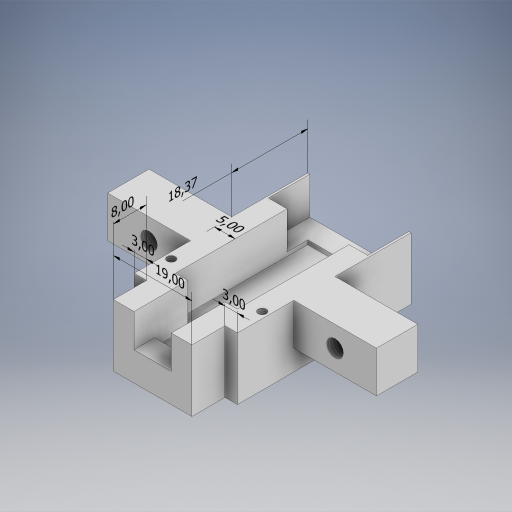
# Autodesk Inventor part: Base
Saved by Autodesk Inventor 2023 (Build 270158000, 158)
## iProperties
Created: 2024-04-01
Part Number: Base
Material: Generic
Document SubType Name: Modeling
Designer: andrew
Density: 1 g/cm^3
Appearance: Default
Author: andrew
Autodesk Inventor part; units mm, degrees
ref_plane "YZ Plane" through (0, 0, 0) normal (1, 0, 0) x (0, 1, 0)
ref_plane "XZ Plane" through (0, 0, 0) normal (0, 1, 0) x (-1, 0, 0)
ref_plane "XY Plane" through (0, 0, 0) normal (0, 0, 1) x (1, 0, 0)
sketch "Sketch1" plane through (0, 0, 0) normal (0, 1, 0) x (-1, 0, 0)
  line L0 (0, 0) -> (15, 0)
  line L1 (15, 0) -> (15, -32)
  line L2 (15, -32) -> (0, -32)
  line L3 (0, -32) -> (0, 0)
  line L4 (3, 0) -> (12, 0)
  line L5 (12, 0) -> (12, 8)
  line L6 (12, 8) -> (3, 8)
  line L7 (3, 8) -> (3, 0)
  line L8 (-5, -32) -> (-5, 5)
  line L9 (-5, 5) -> (-2, 5)
  line L10 (-2, 5) -> (-2, 13)
  line L11 (-2, 13) -> (17, 13)
  line L12 (17, 13) -> (17, 5)
  line L13 (17, 5) -> (20, 5)
  line L14 (20, 5) -> (20, -37)
  line L15 (20, -37) -> (-5, -37)
  line L16 (-5, -37) -> (-5, -32)
  line L17 (-5, -8.634) -> (-25, -8.634)
  line L18 (-25, -8.634) -> (-25, -18.634)
  line L19 (-25, -18.634) -> (-5, -18.634)
  line L20 (-5, -18.634) -> (-5, -8.634)
  line L21 (20, -18.634) -> (40, -18.634)
  line L22 (40, -18.634) -> (40, -8.634)
  line L23 (40, -8.634) -> (20, -8.634)
  line L24 (20, -8.634) -> (20, -18.634)
  dimension "d0" = 15
  dimension "d1" = 32
  dimension "d2" = 9
  dimension "d3" = 3
  dimension "d4" = 3
  dimension "d5" = 8
  dimension "d6" = 5
  dimension "d7" = 5
  dimension "d8" = 5
  dimension "d9" = 5
  dimension "d10" = 5
  dimension "d11" = 5
  dimension "d12" = 5
  dimension "d13" = 5
  dimension "d71" = 20
  dimension "d72" = 10
  dimension "d73" = 20
  dimension "d74" = 10
  constraints: 50 end point, 12 perpendicular, 8 parallel, 4 horizontal, 4 point on line, 1 vertical
  measures "d0" distance of L1.end L2.end
  measures "d1" distance of L0.end L1.end
  measures "d2" distance of L6.end L5.end
  measures "d3" distance between parallel lines of L3 L7
  measures "d4" distance between parallel lines of L1 L5
  measures "d5" distance of L4.end L5.end
  measures "d6" distance between parallel lines of L3 L8
  measures "d7" distance between parallel lines of L2 L15
  measures "d8" distance between parallel lines of L1 L14
  measures "d9" distance between parallel lines of L0 L13
  measures "d10" distance between parallel lines of L5 L12
  measures "d11" distance between parallel lines of L7 L10
  measures "d12" distance between parallel lines of L0 L9
  measures "d13" distance between parallel lines of L6 L11
  measures "d71" distance of L18.end L19.end
  measures "d72" distance of L17.end L18.end
  measures "d73" distance of L21.start L21.end
  measures "d74" distance of L21.end L22.end
extrude "Extrusion1" add sketch "Sketch1" along normal blind 10
sketch "Sketch3" plane through (5, 0, -37) normal (0, 0, -1) x (-1, 0, 0)
  line L0 (0.5, 10) -> (24.5, 10)
  line L1 (24.5, 10) -> (24.5, 1)
  line L2 (24.5, 1) -> (0.5, 1)
  line L3 (0.5, 1) -> (0.5, 10)
  line L4 (25, 0) -> (25, 10) projected
  line L5 (0, 0) -> (0, 10) projected
  line L6 (0, 0) -> (25, 0) projected
  line L7 (0, 10) -> (25, 10) projected
  point P0 (5, 0)
  point P1 (24.5, 5.5)
  dimension "d24" = 0.5
  dimension "d25" = 0.5
  dimension "d26" = 1
  dimension "d27" = 0
  constraints: 8 end point, 2 parallel, 1 horizontal, 1 midpoint, 1 perpendicular
  measures "d24" distance from line of L4 point (24.5, 5.5)
  measures "d25" distance between parallel lines of L5 L3
  measures "d26" distance between parallel lines of L6 L2
  measures "d27" distance between parallel lines of L7 L0
extrude "Extrusion3" cut sketch "Sketch3" against normal blind 10 contours L0 L1 L2 L3
sketch "Sketch4" plane through (-17, 0, 13) normal (0, 0, 1) x (1, 0, 0)
  line L0 (5, 10) -> (14, 10)
  line L1 (14, 10) -> (14, 2)
  line L2 (14, 2) -> (5, 2)
  line L3 (5, 2) -> (5, 10)
  line L4 (0, 0) -> (19, 0) projected
  line L5 (0, 10) -> (19, 10) projected
  line L6 (19, 0) -> (19, 10) projected
  line L7 (0, 0) -> (0, 10) projected
  point P0 (17, 0)
  point P1 (9.5, 0)
  dimension "d30" = 2
  dimension "d31" = 0
  dimension "d32" = 5
  dimension "d33" = 5
  constraints: 8 end point, 2 parallel, 1 horizontal, 1 midpoint, 1 perpendicular
  measures "d30" distance from line of point (9.5, 0) L2
  measures "d31" distance between parallel lines of L5 L0
  measures "d32" distance between parallel lines of L6 L1
  measures "d33" distance between parallel lines of L7 L3
extrude "Extrusion4" cut sketch "Sketch4" against normal blind 10 contours L0 L1 L2 L3
sketch "Sketch5" plane through (0, 0, 0) normal (0, -1, 0) x (1, 0, 0)
  line L0 (-17, 5) -> (-17, 13) projected
  line L1 (2, 13) -> (2, 5) projected
  line L2 (-17, 13) -> (2, 13)
  line L3 (2, 13) -> (2, 5)
  line L4 (5, 5) -> (5, -37) projected
  line L5 (2, 5) -> (5, 5)
  line L6 (5, 5) -> (5, -37)
  line L7 (-20, -37) -> (-20, 5) projected
  line L8 (5, -37) -> (-20, -37)
  line L9 (-20, -37) -> (-20, 5)
  line L10 (-20, 5) -> (-17, 5)
  point P0 (0, 0)
  constraints: 14 end point, 6 perpendicular, 1 horizontal
extrude "Extrusion5" add sketch "Sketch5" along normal blind 5
sketch "Sketch6" plane through (0, 10, 0) normal (0, 1, 0) x (1, 0, 0)
  circle A0 centre (-18.5, 2.5) radius 1
  line L0 (-20, -5) -> (-17, -5) projected
  line L1 (-20, 37) -> (-20, -5) projected
  circle A1 centre (3.5, 2.5) radius 1
  line L2 (2, -5) -> (5, -5) projected
  line L3 (2, -13) -> (2, -5) projected
  point P0 (0, 0)
  dimension "d59" = 2
  dimension "d60" = 7.5
  dimension "d61" = 1.5
  dimension "d62" = 2
  dimension "d63" = 7.5
  dimension "d64" = 1.5
  constraints: 2 centre point
  measures "d59" diameter of A0
  measures "d60" distance from line of A0.centre L0
  measures "d61" distance from line of L1 A0.centre
  measures "d62" diameter of A1
  measures "d63" distance from line of L2 A1.centre
  measures "d64" distance from line of L3 A1.centre
extrude "Extrusion6" cut sketch "Sketch6" against normal blind 5
thread "Thread1" size "M2x0.4" class "6H" standard "ANSI Metric M Profile" full length
thread "Thread2" size "M2x0.4" class "6H" standard "ANSI Metric M Profile" full length
sketch "Sketch7" plane through (25, 0, -18.634) normal (0, 0, -1) x (-1, 0, 0)
  point P0 (25, 0)
sketch "Sketch8" plane through (25, 0, -18.634) normal (0, 0, -1) x (-1, 0, 0)
  circle A0 centre (10, 5) radius 2
  circle A1 centre (55, 5) radius 2
  line L0 (65, 0) -> (65, 10) projected
  line L1 (0, 0) -> (0, 10) projected
  line L2 (0, 10) -> (20, 10) projected
  line L3 (45, 10) -> (65, 10) projected
  point P0 (25, 0)
  point P1 (65, 5)
  dimension "d76" = 4
  dimension "d77" = 4
  dimension "d78" = 10
  dimension "d79" = 10
  dimension "d80" = 5
  dimension "d81" = 5
  constraints: 2 centre point, 1 midpoint
  measures "d76" diameter of A1
  measures "d77" diameter of A0
  measures "d78" distance of point (65, 5) A1.centre
  measures "d79" distance from line of L1 A0.centre
  measures "d80" distance from line of L2 A0.centre
  measures "d81" distance from line of L3 A1.centre
extrude "Extrusion7" cut sketch "Sketch8" against normal blind 10
thread "Thread3" size "M4x0.7" class "6H" standard "ANSI Metric M Profile" full length
thread "Thread4" size "M4x0.7" class "6H" standard "ANSI Metric M Profile" full length
body "Solid1" dims "d1" = 32
